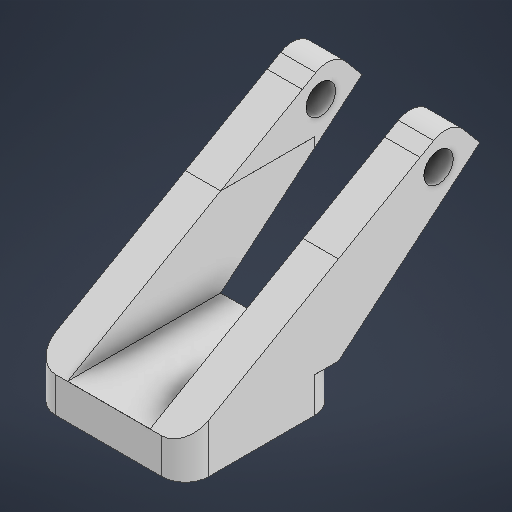
# Autodesk Inventor part: PodstawkaKola Próba 1
Saved by Autodesk Inventor 2026 (Build 300175000, 175)
## iProperties
Created: 2025-04-29
Part Number: PodstawkaKola Próba 1
Material: Generic
Document SubType Name: Modeling
Designer: isan
Density: 1 g/cm^3
Appearance: Default
Author: isan
Autodesk Inventor part; units mm, degrees
ref_plane "YZ Plane" through (0, 0, 0) normal (1, 0, 0) x (0, 1, 0)
ref_plane "XZ Plane" through (0, 0, 0) normal (0, 1, 0) x (-1, 0, 0)
ref_plane "XY Plane" through (0, 0, 0) normal (0, 0, 1) x (1, 0, 0)
sketch "Sketch1" plane through (0, 0, 0) normal (0, 0, 1) x (1, 0, 0)
  line L0 (6.5, 6.5) -> (-6.5, 6.5)
  line L1 (-6.5, 6.5) -> (-6.5, -6.5)
  line L2 (-6.5, -6.5) -> (6.5, -6.5)
  line L3 (6.5, -6.5) -> (6.5, 6.5)
  line L4 (6.5, 6.5) -> (-6.5, -6.5) construction
  line L5 (-6.5, 6.5) -> (6.5, -6.5) construction
  point P0 (0, 0)
  point P1 (0, 0)
  dimension "d35" = 13
  dimension "d36" = 13
  constraints: 12 end point, 2 parallel, 1 coincident, 1 horizontal, 1 midpoint, 1 perpendicular
  measures "d35" distance of L1.end L2.end
  measures "d36" distance of L0.end L1.end
extrude "Extrusion1" add sketch "Sketch1" along normal blind 3
sketch "Sketch2" plane through (0, 0, 0) normal (0, 0, -1) x (-1, 0, 0)
  line L0 (-6.5, 1) -> (6.5, 1)
  line L1 (6.5, 1) -> (6.5, -1)
  line L2 (6.5, -1) -> (-6.5, -1)
  line L3 (-6.5, -1) -> (-6.5, 1)
  line L4 (-6.5, 1) -> (6.5, -1) construction
  line L5 (6.5, 1) -> (-6.5, -1) construction
  circle A0 centre (0, 0) radius 4.9
  point P0 (4.7969, 1)
  point P1 (-4.7969, 1)
  point P2 (-4.7969, -1)
  point P3 (4.7969, -1)
  dimension "d3" = 2
  dimension "d4" = 13
  dimension "d57" = 9.8
  constraints: 12 end point, 2 midpoint, 2 parallel, 1 centre point, 1 coincident, 1 horizontal, 1 perpendicular
  measures "d3" distance of L0.end L1.end
  measures "d4" distance of L1.end L2.end
  measures "d57" diameter of A0
extrude "Extrusion2" cut sketch "Sketch2" against normal blind 1.1 contours L0 A0 L2
sketch "Sketch6" plane through (0, 0, 3) normal (0, 0, 1) x (1, 0, 0)
  line L0 (3.5, 6.5) -> (6.5, 6.5)
  line L1 (6.5, 6.5) -> (6.5, -6.5)
  line L2 (6.5, -6.5) -> (3.5, -6.5)
  line L3 (3.5, -6.5) -> (3.5, 6.5)
  line L4 (3.5, 6.5) -> (6.5, -6.5) construction
  line L5 (6.5, 6.5) -> (3.5, -6.5) construction
  line L6 (-3.5, 6.5) -> (-6.5, 6.5)
  line L7 (-6.5, 6.5) -> (-6.5, -6.5)
  line L8 (-6.5, -6.5) -> (-3.5, -6.5)
  line L9 (-3.5, -6.5) -> (-3.5, 6.5)
  line L10 (-3.5, 6.5) -> (-6.5, -6.5) construction
  line L11 (-6.5, 6.5) -> (-3.5, -6.5) construction
  line L12 (10.9648, 0) -> (-10.9648, 0) construction
  point P0 (0, 0)
  point P1 (5, 0)
  point P2 (-5, 0)
  point P3 (0, 0)
  dimension "d29" = 5
  dimension "d30" = 5
  dimension "d31" = 3
  dimension "d32" = 3
  dimension "d33" = 13
  dimension "d34" = 13
  constraints: 26 end point, 5 midpoint, 4 parallel, 3 horizontal, 2 perpendicular, 2 point on line, 1 coincident
  measures "d29" distance of point (0, 0) point (5, 0)
  measures "d30" distance of point (0, 0) point (-5, 0)
  measures "d31" distance of L7.end L8.end
  measures "d32" distance of L1.end L2.end
  measures "d33" distance of L0.end L1.end
  measures "d34" distance of L6.end L7.end
extrude "Extrusion6" add sketch "Sketch6" along normal blind 7.5
chamfer "Chamfer5" distance 13 angle 30 1 edges at (-5, -6.5, 10.5) measured on face at (-4.5, -2.1667, 10.5)
sketch "Sketch10" plane through (-6.5, 6.5, 0) normal (0, 1, 0) x (1, 0, 0)
  line L0 (3, -10.5) -> (0, -10.5) projected
  line L1 (0, -10.5) -> (0, -2.9944) projected
  line L2 (3, -10.5) -> (0, -10.5)
  line L3 (0, -10.5) -> (0, -2.9944)
  line L4 (0, -2.9944) -> (3, -2.9944)
  line L5 (3, -2.9944) -> (3, -10.5)
  line L6 (10, -10.5) -> (10, -3) projected
  line L7 (13, 0) -> (13, -2.9944) projected
  line L8 (10, -10.5) -> (13, -10.5)
  line L9 (13, -10.5) -> (13, -2.9944)
  line L10 (13, -2.9944) -> (10, -2.9944)
  line L11 (10, -2.9944) -> (10, -10.5)
  point P0 (6.5, 0)
  constraints: 16 end point, 4 parallel, 2 horizontal, 2 perpendicular
extrude "Extrusion10" add sketch "Sketch10" along normal blind 8
chamfer "Chamfer6" distance 6.712 angle 50 1 edges at (-5, 14.5, 2.9944) measured on face at (-5.5, 14.5, 7.9981)
chamfer "Chamfer7" distance 6.712 angle 50 1 edges at (5, 14.5, 2.9944) measured on face at (5.5, 14.5, 5.4981)
sketch "Sketch16" plane through (3.5, 6.5, 10.5) normal (0, 0, 1) x (1, 0, 0)
  line L0 (3, 8) -> (3, 0.0009) projected
  line L1 (0, 0) -> (0, 8) projected
  line L2 (3, 0.0009) -> (0, 0.0009)
  line L3 (0, 0.0009) -> (0, 8)
  line L4 (0, 8) -> (3, 8)
  line L5 (3, 8) -> (3, 0.0009)
  line L6 (-10, 0) -> (-10, -13) projected
  line L7 (-6.9951, 8) -> (-10, 8)
  line L8 (-10, 8) -> (-10, 0)
  line L9 (-10, 0) -> (-6.9951, 0)
  line L10 (-6.9951, 0) -> (-6.9951, 8)
  point P0 (-3.5, -6.5)
  point P1 (0, 0.0009)
  constraints: 16 end point, 4 parallel, 2 horizontal, 2 perpendicular, 1 point on line
extrude "Extrusion14" add sketch "Sketch16" along normal blind 4
chamfer "Chamfer11" distance 6.928 angle 30 1 edges at (5, 6.5009, 14.5) measured on face at (4.5, 11.8336, 14.5)
chamfer "Chamfer12" distance 6.928 angle 30 1 edges at (-4.9975, 6.5, 14.5) measured on face at (-4.4967, 9.1667, 14.5)
sketch "Sketch17" plane through (-6.5, 14.5, 0) normal (0, 1, 0) x (1, 0, 0)
  line L0 (0, -9.7064) -> (3, -9.7064) projected
  line L1 (3.0049, -14.5) -> (0, -14.5) projected
  line L2 (0, -9.7064) -> (3.0049, -9.7064)
  line L3 (3.0049, -9.7064) -> (3.0049, -14.5)
  line L4 (3.0049, -14.5) -> (0, -14.5)
  line L5 (0, -14.5) -> (0, -9.7064)
  line L6 (10, -14.5) -> (10, -10.5001) projected
  line L7 (13, -9.7064) -> (13, -2.9944) projected
  line L8 (10, -14.5) -> (13, -14.5)
  line L9 (13, -14.5) -> (13, -9.7064)
  line L10 (13, -9.7064) -> (10, -9.7064)
  line L11 (10, -9.7064) -> (10, -14.5)
  point P0 (6.5, 0)
  constraints: 16 end point, 4 parallel, 2 horizontal, 2 perpendicular
extrude "Extrusion15" add sketch "Sketch17" along normal blind 4
chamfer "Chamfer13" distance 3.355 angle 50 1 edges at (5, 18.5, 9.7064) measured on face at (4.5, 18.5, 11.3043)
chamfer "Chamfer14" distance 3.355 angle 50 1 edges at (-4.9975, 18.5, 9.7064) measured on face at (-5.4984, 18.5, 11.3043)
sketch "Sketch18" plane through (-6.5, 18.5, 0) normal (0, 1, 0) x (1, 0, 0)
  line L0 (0, -14.5) -> (0, -10.5001) projected
  line L1 (0, -13.0614) -> (3.0049, -13.0614) projected
  line L2 (0, -14.5) -> (3.0049, -14.5)
  line L3 (3.0049, -14.5) -> (3.0049, -13.0614)
  line L4 (3.0049, -13.0614) -> (0, -13.0614)
  line L5 (0, -13.0614) -> (0, -14.5)
  line L6 (13, -10.5001) -> (13, -14.5) projected
  line L7 (10, -14.5) -> (10, -10.5001) projected
  line L8 (13, -14.5) -> (10, -14.5)
  line L9 (10, -14.5) -> (10, -13.0614)
  line L10 (10, -13.0614) -> (13, -13.0614)
  line L11 (13, -13.0614) -> (13, -14.5)
  point P0 (6.5, 0)
  constraints: 16 end point, 4 parallel, 2 horizontal, 2 perpendicular, 2 point on line
extrude "Extrusion16" add sketch "Sketch18" along normal blind 1.5
chamfer "Chamfer15" distance 1.258 angle 50 1 edges at (5, 20, 13.0614) measured on face at (4.5, 20, 14.0205)
chamfer "Chamfer16" distance 1.258 angle 50 1 edges at (-4.9975, 20, 13.0614) measured on face at (-5.4984, 20, 13.541)
sketch "Sketch19" plane through (6.5, -6.5, 0) normal (1, 0, 0) x (0, 0, -1)
  circle A0 centre (-13, 21.5) radius 1.25
  line L0 (0, 0) -> (0, 13) projected
  point P0 (0, 6.5)
  point P1 (0, 6.5)
  point P2 (0, 6.5)
  dimension "d114" = 2.5
  dimension "d115" = 15
  dimension "d116" = 13
  constraints: 2 midpoint, 1 centre point
  measures "d114" diameter of A0
  measures "d115" vertical distance of point (0, 6.5) A0.centre
  measures "d116" horizontal distance of A0.centre point (0, 6.5)
extrude "Extrusion17" cut sketch "Sketch19" against normal blind 13
sketch "Sketch20" plane through (3.5, 6.5, 14.5) normal (0, 0, 1) x (1, 0, 0)
  line L0 (3, 0.0009) -> (3, 6.9289) projected
  line L1 (3, 6.9289) -> (0, 6.9289)
  line L2 (0, 6.9289) -> (0, 13.5)
  line L3 (0, 13.5) -> (3, 13.5)
  line L4 (3, 13.5) -> (3, 6.9289)
  line L5 (-6.9951, 0) -> (-6.9951, 8) projected
  line L6 (-6.9951, 6.9289) -> (-9.9959, 6.9289)
  line L7 (-9.9959, 6.9289) -> (-9.9959, 13.5)
  line L8 (-9.9959, 13.5) -> (-6.9951, 13.5)
  line L9 (-6.9951, 13.5) -> (-6.9951, 6.9289)
  point P0 (-3.5, -6.5)
  constraints: 16 end point, 4 parallel, 3 point on line, 2 horizontal, 2 perpendicular
extrude "Extrusion18" add sketch "Sketch20" along normal blind 2
chamfer "Chamfer17" distance 3.464 angle 30 1 edges at (5, 13.4289, 16.5) measured on face at (4.5, 17.8096, 16.5)
chamfer "Chamfer18" distance 3.464 angle 30 1 edges at (-4.9955, 13.4289, 16.5) measured on face at (-5.4956, 17.8096, 16.5)
sketch "Sketch21" plane through (6.5, -6.5, 0) normal (1, 0, 0) x (0, 0, -1)
  line L0 (-14.5001, 19.9289) -> (-16.5, 23.3929) projected
  line L1 (-13.0614, 25) -> (-9.7064, 21.0017) projected
  line L2 (-16.0029, 22.5319) -> (-13.0614, 25)
  line L3 (-13.0614, 25) -> (-15.218, 28.5486)
  line L4 (-15.218, 28.5486) -> (-18.5529, 25)
  line L5 (-18.5529, 25) -> (-17.0876, 20.6155)
  line L6 (-17.0876, 20.6155) -> (-16.0029, 22.5319)
  point P0 (0, 6.5)
  constraints: 10 end point, 1 perpendicular, 1 point on line
extrude "Extrusion19" cut sketch "Sketch21" against normal blind 13
fillet "Fillet4" radius 2 2 edges at (5, 16.0319, 16.0029) (-4.9955, 16.0319, 16.0029)
fillet "Fillet5" radius 2 4 edges at (-6.5, -6.5, 1.4975) (-6.5, 6.5, 1.4972) (6.5, 6.5, 1.4972) (6.5, -6.5, 1.4975)
body "Solid1"
